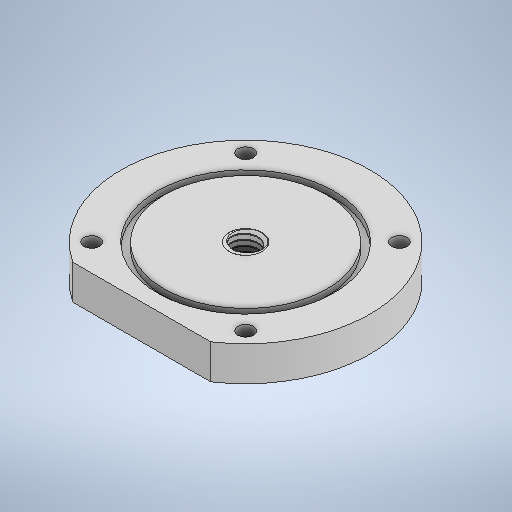
# Autodesk Inventor part: Access Cap
Saved by Autodesk Inventor 2025 (Build 290162000, 162)
## iProperties
Created: 2025-10-23
Part Number: Access Cap
Material: Generic
Document SubType Name: Modeling
Designer: mumin
Density: 1 g/cm^3
Appearance: Default
Author: mumin
Autodesk Inventor part; units mm, degrees
ref_plane "YZ Plane" through (0, 0, 0) normal (1, 0, 0) x (0, 1, 0)
ref_plane "XZ Plane" through (0, 0, 0) normal (0, 1, 0) x (-1, 0, 0)
ref_plane "XY Plane" through (0, 0, 0) normal (0, 0, 1) x (1, 0, 0)
sketch "Sketch1" plane through (0, 0, 0) normal (0, 1, 0) x (-1, 0, 0)
  circle A0 centre (0, 0) radius 36
  line L0 (19.8997, 30) -> (-19.8997, 30)
  dimension "d0" = 72
  dimension "d1" = 30
  constraints: 2 end point, 2 point on circle, 1 centre point, 1 coincident, 1 horizontal
  measures "d0" diameter of A0
  measures "d1" distance from line of point (0, 0) L0
extrude "Base" add sketch "Sketch1" along normal blind 10 contours A0 L0 picked at (-0.4083, 8.0069)
sketch "Sketch2" plane through (0, 0, 0) normal (0, -1, 0) x (1, 0, 0)
  circle A0 centre (0, 0) radius 31.4
  line L0 (22.2032, 22.2032) -> (0, 0)
  line L1 (-50.4, 0) -> (50.4, 0) projected
  dimension "d11" = 62.8
  dimension "d12" = 45
  constraints: 2 end point, 1 coincident, 3 other
  measures "d12" angle of L1 L0
hole "Mounting Holes" at (22.2032, 0, 22.2032) direction (0, 1, 0) diameter 4.5 end through all counterbore diameter 8 counterbore depth 4
pattern_circular "Circular Pattern1" count 4 over 360 about axis through (0, 0, 0) along (0, 1, 0) of "Mounting Holes"
sketch "Sketch3" plane through (0, 0, 0) normal (0, 0, 1) x (1, 0, 0)
  line L0 (36, 10) -> (-36, 10) projected
  line L1 (-25.5, 10) -> (-23.5, 10)
  line L2 (-23.5, 10) -> (-23.5, 8.2)
  line L3 (-23.5, 8.2) -> (-25.5, 8.2)
  line L4 (-25.5, 8.2) -> (-25.5, 10)
  line L5 (0, -2) -> (0, 12) projected
  point P0 (0, 0)
  point P1 (19.8997, 10)
  point P2 (-19.8997, 10)
  point P3 (0, 10)
  dimension "d16" = 2
  dimension "d17" = 1.8
  dimension "d18" = 23.5
  constraints: 8 end point, 2 parallel, 1 horizontal, 1 midpoint, 1 perpendicular, 1 point on line
  measures "d16" distance of L2.end L3.end
  measures "d17" distance of L1.end L2.end
  measures "d18" distance from line of point (0, 10) L2
revolve "Seal Groove" cut sketch "Sketch3" angle 360 about axis through (0, -10, 0) along (0, 1, 0)
sketch "Sketch4" plane through (0, 0, 0) normal (0, -1, 0) x (1, 0, 0)
  point P0 (0, 0)
  point P1 (0, 0)
  constraints: 1 coincident
hole "Wire Passthrough" at (0, 0, 0) direction (0, 1, 0) diameter 9.5 end through all
thread "Thread3" size "M10x1.5" class "6H" standard "ANSI Metric M Profile" length 10
sketch "Sketch14" plane through (0, 10, 0) normal (1, 0, 0) x (0, 0, 1)
  line L0 (4.75, 0) -> (4.75, 10)
  line L1 (4.75, 10) -> (3.6378, 10)
  line L2 (3.6378, 10) -> (3.6378, 0)
  line L3 (3.6378, 0) -> (4.75, 0)
  line L4 (0, -3.9629) -> (0, 12.3271) projected
  constraints: 8 end point
revolve "Revolution5" add sketch "Sketch14" angle 360 about axis through (0, 10, 0) along (0, -1, 0) separate body
sketch "Sketch13" plane through (0, 10, 4.75) normal (-1, 0, 0) x (0, -1, 0)
  line L0 (-0.8751, -0.076) -> (-0.7501, -0.076) construction
  line L1 (0.1249, -1.0365) -> (-0.0001, -1.2766) construction
  line L2 (-1.5001, -1.2766) -> (-1.6251, -1.0365) construction
  line L3 (-0.6251, -0.076) -> (-0.7501, 0.1641) construction
  line L4 (-0.7501, 0.1641) -> (-0.8751, -0.076) construction
  line L5 (-1.5001, -1.2766) -> (-1.3751, -1.0365) construction
  line L6 (-0.6251, -0.076) -> (-0.1251, -1.0365)
  line L7 (-1.6251, -1.0365) -> (-1.3751, -1.0365) construction
  arc A0 (-1.6251, -1.0365) -> (-1.5001, -1.1124) centre (-1.5001, -0.9714) ccw construction
  line L8 (0.1249, -1.0365) -> (-0.1251, -1.0365) construction
  line L9 (-1.5001, -1.2766) -> (-1.5001, -1.0365) construction
  line L10 (-0.0001, -1.2766) -> (-0.0001, -1.0365) construction
  line L11 (-0.7501, 0.1641) -> (-0.7501, -0.0002) construction
  line L12 (-1.5001, -1.1124) -> (-0.0001, -1.1124)
  arc A1 (-1.5001, -1.1124) -> (-1.3751, -1.0365) centre (-1.5001, -0.9714) ccw
  line L13 (-0.1251, -1.0365) -> (-0.0001, -1.2766) construction
  line L14 (-1.3751, -1.0365) -> (-0.8751, -0.076)
  line L15 (-0.0001, -0.0002) -> (-0.0001, 0.0177)
  line L16 (-0.0001, 0.0177) -> (-0.0001, -0.0002)
  line L17 (-0.0001, -0.0002) -> (0.0334, -0.0002)
  arc A2 (-0.1251, -1.0365) -> (-0.0001, -1.1124) centre (-0.0001, -0.9714) ccw
  arc A3 (-0.0001, -1.1124) -> (0.1249, -1.0365) centre (-0.0001, -0.9714) ccw construction
  arc A4 (-0.7501, -0.0002) -> (-0.8751, -0.076) centre (-0.7501, -0.1411) ccw
  arc A5 (-0.6251, -0.076) -> (-0.7501, -0.0002) centre (-0.7501, -0.1411) ccw
  line L18 (-0.7501, -0.0002) -> (-0.7501, -0.076) construction
  line L19 (-0.7501, -0.076) -> (-0.6251, -0.076) construction
  dimension "d87" = 55
  dimension "d88" = 0.2401
  dimension "d89" = 0.2401
  dimension "Sketch13_ThreadOffset" = 0
  dimension "Sketch13_MajorRadius" = 1.1122
  dimension "d92" = 1.5
  dimension "Sketch13_MinorRadius" = 0
  constraints: 40 end point, 12 point on circle, 10 parallel, 8 tangent, 6 centre point, 6 collinear, 2 midpoint, 2 point on line, 1 horizontal, 1 perpendicular, 3 other
  measures "d87" angle of L6 L14
  measures "d88" distance of L3.end L0.end
  measures "d89" distance of L1.end L10.end
  measures "Sketch13_ThreadOffset" distance between parallel lines of L15 L10
  measures "Sketch13_MajorRadius" distance from line of L12 L15.start
  measures "d92" distance from line of L1.end L9
  measures "Sketch13_MinorRadius" distance edge to line of A5 L17
coil "Coil4" sketch "Sketch13" operation cut axis through (0, 10, 0) along (0, -1, 0) pitch 1.5015 turns 8.658009 hand right bodies 2
equation "\"d87\" = d94"
equation "\"d88\" = 0.160083 * Sketch13_Pitch"
equation "\"d89\" = 0.160083 * Sketch13_Pitch"
equation "\"d92\" = Sketch13_Pitch"
equation "\"d36\" = 55deg"
equation "\"Sketch5_Pitch\" = 1.25"
equation "\"d54\" = 55deg"
equation "\"Sketch7_Pitch\" = 1.25"
equation "\"d74\" = 55deg"
equation "\"Sketch10_Pitch\" = 1.5"
equation "\"d94\" = 55deg"
equation "\"Sketch13_Pitch\" = 1.5"
body "Solid1"
body "Solid5"
